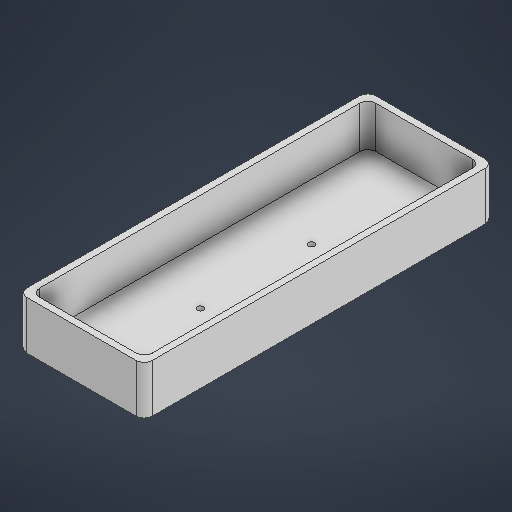
# Autodesk Inventor part: Kepala
Saved by Autodesk Inventor 2026.2 (Build 302298010, 298A)
## iProperties
Created: 2026-05-16
Part Number: Kepala
Material: Generic
Document SubType Name: Modeling
Designer: Martina
Density: 1 g/cm^3
Appearance: Default
Author: Martina
Autodesk Inventor part; units mm, degrees
ref_plane "YZ Plane" through (0, 0, 0) normal (1, 0, 0) x (0, 1, 0)
ref_plane "XZ Plane" through (0, 0, 0) normal (0, 1, 0) x (-1, 0, 0)
ref_plane "XY Plane" through (0, 0, 0) normal (0, 0, 1) x (1, 0, 0)
sketch "Sketch1" plane through (0, 0, 0) normal (0, 1, 0) x (-1, 0, 0)
  line L0 (5, 0) -> (73, 0)
  line L1 (78, -5) -> (78, -212)
  line L2 (73, -217) -> (5, -217)
  line L3 (0, -212) -> (0, -5)
  line L4 (69, -4) -> (9, -4)
  line L5 (4, -9) -> (4, -208)
  line L6 (9, -213) -> (69, -213)
  line L7 (74, -208) -> (74, -9)
  line L8 (74, -4) -> (4, -213) construction
  line L9 (4, -4) -> (74, -213) construction
  arc A0 (78, -5) -> (73, 0) centre (73, -5) ccw
  arc A1 (5, 0) -> (0, -5) centre (5, -5) ccw
  arc A2 (73, -217) -> (78, -212) centre (73, -212) ccw
  arc A3 (0, -212) -> (5, -217) centre (5, -212) ccw
  arc A4 (74, -9) -> (69, -4) centre (69, -9) ccw
  arc A5 (9, -4) -> (4, -9) centre (9, -9) ccw
  arc A6 (69, -213) -> (74, -208) centre (69, -208) ccw
  arc A7 (4, -208) -> (9, -213) centre (9, -208) ccw
  circle A8 centre (39, -143) radius 2
  line L10 (39, -108.5) -> (37, -108.5)
  circle A9 centre (39, -74) radius 2
  point P0 (0, 0)
  point P1 (78, -217)
  point P2 (78, 0)
  point P3 (0, -217)
  dimension "d0" = 78
  dimension "d1" = 217
  dimension "d2" = 70
  dimension "d3" = 209
  dimension "d4" = 5
  dimension "d5" = 5
  dimension "d10" = 4
  dimension "d14" = 69
  constraints: 22 end point, 16 point on circle, 16 point on line, 16 tangent, 10 centre point, 6 equal radius, 4 parallel, 3 horizontal, 2 midpoint, 2 perpendicular, 1 symmetric about line, 1 other
  measures "d0" distance of point (78, -217) point (0, -217)
  measures "d1" distance of point (78, 0) point (78, -217)
  measures "d2" distance of L9.end L8.end
  measures "d3" distance of L8.end L9.start
  measures "d4" radius of A0
  measures "d5" radius of A4
  measures "d10" diameter of A8
  measures "d14" distance of A9.centre A8.centre
extrude "Extrusion1" add sketch "Sketch1" along normal blind 30 contours L0 A0 L1 A2 L2 A3 L3 A1
extrude "Extrusion2" add sketch "Sketch1" along normal blind 4 contours A4 L7 A6 L6 A7 L5 A5 L4 | A8 | A9
extrude "Extrusion3" cut sketch "Sketch1" along normal blind 4 contours A8 | A9
body "Solid1"
